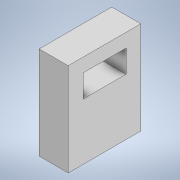
# Autodesk Inventor part: SecondaryBracket
Saved by Autodesk Inventor 2021 (Build 250183000, 183)
## iProperties
Created: 2022-01-19
Part Number: SecondaryBracket
Material: Generic
Document SubType Name: Modeling
Designer: Tlar613
Density: 1 g/cm^3
Appearance: Default
Author: Tlar613
Autodesk Inventor part; units mm, degrees
ref_plane "YZ Plane" through (0, 0, 0) normal (1, 0, 0) x (0, 1, 0)
ref_plane "XZ Plane" through (0, 0, 0) normal (0, 1, 0) x (-1, 0, 0)
ref_plane "XY Plane" through (0, 0, 0) normal (0, 0, 1) x (1, 0, 0)
sketch "Sketch1" plane through (0, 0, 0) normal (1, 0, 0) x (0, 1, 0)
  line L0 (0, 0) -> (32, 0)
  line L1 (32, 0) -> (32, 25)
  line L2 (32, 25) -> (0, 25)
  line L3 (0, 25) -> (0, 0)
  line L4 (27.3, 19.9) -> (19.5, 19.9)
  line L5 (19.5, 19.9) -> (19.5, 5.1)
  line L6 (19.5, 5.1) -> (27.3, 5.1)
  line L7 (27.3, 5.1) -> (27.3, 19.9)
  dimension "d0" = 32
  dimension "d1" = 25
  dimension "d2" = 14.8
  dimension "d3" = 7.8
  dimension "d4" = 5.1
  dimension "d5" = 19.5
  constraints: 16 end point, 4 parallel, 2 horizontal, 2 perpendicular
  measures "d0" distance of L1.end L2.end
  measures "d1" distance of L0.end L1.end
  measures "d2" distance of L6.end L4.start
  measures "d3" distance of L4.start L4.end
  measures "d4" distance between parallel lines of L2 L4
  measures "d5" distance between parallel lines of L3 L5
extrude "Extrusion1" add sketch "Sketch1" along normal blind 10
body "Solid1"
